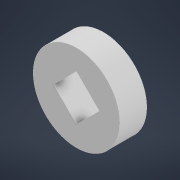
# Autodesk Inventor part: 7
Saved by Autodesk Inventor 2021.2 (Build 252289000, 289)
## iProperties
Created: 2023-09-06
Part Number: 7
Material: Типовые
Document SubType Name: Modeling
Designer: User
Density: 1 g/cm^3
Appearance: По умолчанию
Author: User
Autodesk Inventor part; units mm, degrees
ref_plane "YZ Plane" through (0, 0, 0) normal (1, 0, 0) x (0, 1, 0)
ref_plane "XZ Plane" through (0, 0, 0) normal (0, 1, 0) x (-1, 0, 0)
ref_plane "XY Plane" through (0, 0, 0) normal (0, 0, 1) x (1, 0, 0)
sketch "Эскиз1" plane through (0, 0, 0) normal (0, 0, 1) x (1, 0, 0)
  circle A0 centre (0, 0) radius 16
  line L0 (0, 8.4853) -> (8.4853, 0)
  line L1 (8.4853, 0) -> (0, -8.4853)
  line L2 (0, -8.4853) -> (-8.4853, 0)
  line L3 (-8.4853, 0) -> (0, 8.4853)
  dimension "d0" = 32
  dimension "d1" = 12
  constraints: 8 end point, 2 coincident, 1 centre point, 9 other
  measures "d0" diameter of A0
  measures "d1" distance of L2.end L0.start
extrude "Выдавливание1" add sketch "Эскиз1" along normal mid plane 10
